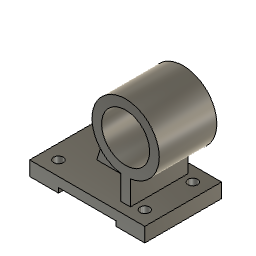
A2_AI22BTECH11005_5 (Autodesk Fusion 360 design; units mm, degrees)
Autodesk Fusion 360 part; units mm, degrees
sketch "Sketch1" plane through (0, 0, 0) normal (0, 1, 0) x (1, 0, 0)
  line L0 (0, 0) -> (60, 0)
  line L1 (0, 0) -> (-60, 0)
  line L2 (-60, 0) -> (-60, 15)
  line L3 (-60, 15) -> (-40, 15)
  line L4 (30, 10) -> (-30, 10)
  line L5 (40, 15) -> (60, 15)
  line L6 (60, 15) -> (60, 0)
  line L7 (-40, 15) -> (-30, 15)
  line L8 (-30, 15) -> (-30, 10)
  line L9 (30, 10) -> (30, 15)
  line L10 (40, 15) -> (30, 15)
  line L11 (60, 0) -> (30, 0)
  line L12 (30, 0) -> (35, 0)
  line L13 (35, 0) -> (25, 0)
  line L14 (25, 0) -> (25, -25.359)
  line L15 (35, -25.359) -> (35, 0)
  arc A0 (25, -25.359) -> (35, -25.359) centre (30, -60) ccw
  circle A1 centre (30, -60) radius 25
  line L16 (25, 0) -> (-30, 0)
  line L17 (-60, 0) -> (-25, 0)
  line L18 (-25, 0) -> (-3.4631, -70.2578)
  constraint coincident L0.start L1.start
  constraint horizontal L0
  constraint parallel L0 L1
  constraint perpendicular L1 L2
  constraint perpendicular L2 L3
  constraint perpendicular L0 L6
  constraint perpendicular L4 L8
  constraint perpendicular L4 L9
  constraint perpendicular L9 L10
  constraint midpoint L0 L11.end
  constraint coincident L11 L12.end
  constraint perpendicular L6 L12
  constraint coincident L0 L13.end
  constraint parallel L0 L13
  constraint perpendicular L13 L14
  constraint perpendicular L0 L15
  constraint concentric A0 A1
  constraint midpoint L1 L16.end
  constraint coincident L16 L17.end
  constraint perpendicular L2 L17
  constraint coincident A0 L18.end
  constraint tangent A0 L18
extrude "Extrude1" add sketch "Sketch1" along normal blind 40 contours L0 L1 L2 L3 L4 L5 L6 L7 L8 L9 L10 L11 L12 L13 L16 L17
extrude "Extrude3" add sketch "Sketch1" along normal blind 30 contours L0 L11 L12 L13 L14 L15 A0
extrude "Extrude2" add sketch "Sketch1" along normal blind 5 contours L0 L1 L14 A0 L16 L18
sketch "Sketch2" plane through (0, 0, 0) normal (0, 0, 1) x (-1, 0, 0)
  line L0 (25, -5) -> (-25, -5)
  line L1 (-25, -5) -> (-25, -30)
  line L2 (-25, -30) -> (-35, -30)
  line L3 (-35, -30) -> (-35, 0)
  line L4 (-35, 0) -> (-60, 0)
  line L5 (-60, 0) -> (-60, -40)
  line L6 (-60, -40) -> (60, -40)
  line L7 (60, -40) -> (60, 0)
  line L8 (60, 0) -> (25, 0)
  line L9 (25, 0) -> (25, -5)
  line L10 (-60, -40) -> (-45, -40)
  line L11 (-45, -40) -> (-45, -25)
  circle A0 centre (-45, -25) radius 5
  line L12 (60, -40) -> (60, -25)
  line L13 (60, -25) -> (45, -25)
  circle A1 centre (45, -25) radius 5
  dimension "d7" = 10
  dimension "d8" = 10
  constraint coincident L5.end L6.start
  constraint coincident L6 L10.end
  constraint perpendicular L5 L10
  constraint perpendicular L6 L11
  constraint coincident L11.end A0.centre
  constraint coincident L6.end L7.start
  constraint coincident L7 L12.end
  constraint perpendicular L6 L12
  constraint perpendicular L7 L13
  constraint coincident L13.end A1.centre
  measures "d7" diameter of A0
  measures "d8" diameter of A1
extrude "Extrude4" cut sketch "Sketch2" against normal blind 15 contours A0 | A1
mirror "Mirror1" about plane through (0, 0, 0) normal (0, -1, 0) of bodies 1 merged
